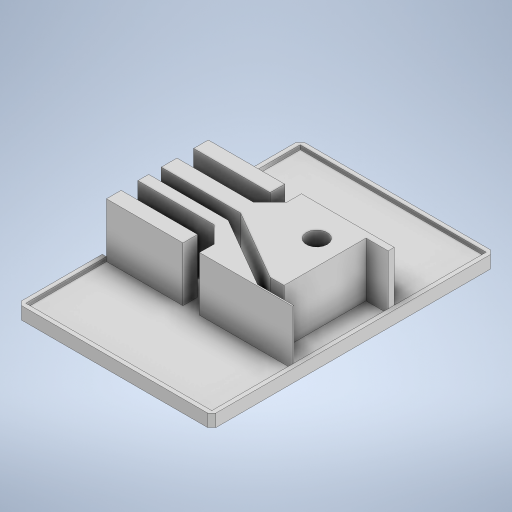
# Autodesk Inventor part: Suporte
Saved by Autodesk Inventor 2024 (Build 280153020, 153B)
## iProperties
Created: 2023-05-31
Part Number: Suporte
Material: Genérico
Document SubType Name: Modeling
Designer: victo
Density: 1 g/cm^3
Appearance: Padrão
Author: victo
Autodesk Inventor part; units mm, degrees
ref_plane "YZ Plane" through (0, 0, 0) normal (1, 0, 0) x (0, 1, 0)
ref_plane "XZ Plane" through (0, 0, 0) normal (0, 1, 0) x (-1, 0, 0)
ref_plane "XY Plane" through (0, 0, 0) normal (0, 0, 1) x (1, 0, 0)
sketch "Esboço1" plane through (0, 0, 0) normal (0, 1, 0) x (-1, 0, 0)
  line L0 (0.0003, 60.0007) -> (0.0003, 29.9998)
  line L1 (0.0003, 29.9998) -> (0.0003, 29.9999)
  line L2 (-0.9997, 29.9999) -> (-0.9997, 60.0007)
  circle A0 centre (11.1, 41.2) radius 2.5
  line L3 (5.3003, 54.8257) -> (5.3003, 35.2257)
  line L4 (5.3003, 35.2257) -> (0.0003, 35.2257)
  line L5 (0.0003, 29.9999) -> (0.0003, 14.4635)
  line L6 (-0.9997, 14.4635) -> (-0.9997, 29.9999)
  line L7 (44.5003, 33.7635) -> (45.5003, 33.7635)
  line L8 (44.5003, 58.1254) -> (45.5003, 58.1254)
  line L9 (26.2003, 33.7635) -> (26.2003, 37.2635)
  line L10 (26.2003, 37.2635) -> (44.5003, 37.2635)
  line L11 (22.2003, 33.7635) -> (0.0003, 33.7635)
  line L12 (22.2003, 33.7635) -> (22.2003, 37.2635)
  line L13 (26.2003, 33.7635) -> (45.0003, 33.7635)
  line L14 (37.268, 41.2635) -> (44.5003, 41.2635)
  line L15 (22.2003, 37.2635) -> (26.2003, 41.2635)
  line L16 (37.268, 41.2635) -> (26.2003, 41.2635)
  line L17 (43.0622, 54.6254) -> (44.5003, 54.6254)
  line L18 (43.0622, 54.6254) -> (26.2003, 54.6254)
  line L19 (26.2003, 54.6254) -> (26.2003, 58.1254)
  line L20 (22.2003, 54.6254) -> (22.2503, 58.1254)
  line L21 (26.2003, 50.6254) -> (22.2003, 54.6254)
  line L22 (26.2003, 50.6254) -> (44.5003, 50.6254)
  line L23 (5.3003, 54.8257) -> (8.6381, 54.8257)
  line L24 (8.6381, 57.8257) -> (0.0003, 57.8257)
  line L25 (44.5003, 45.0257) -> (25.488, 45.0257)
  line L26 (25.488, 48.0257) -> (44.5003, 48.0257)
  line L27 (8.6381, 57.8257) -> (25.488, 48.0257)
  line L28 (8.6381, 54.8257) -> (25.488, 45.0257)
  line L29 (0.0003, 58.1254) -> (22.2503, 58.1254)
  line L30 (26.2003, 58.1254) -> (44.5003, 58.1254)
  line L31 (44.5003, 54.6254) -> (44.5003, 58.1254)
  line L32 (44.5003, 48.0257) -> (44.5003, 50.6254)
  line L33 (44.5003, 33.7635) -> (44.5003, 37.2635)
  line L34 (44.5003, 41.2635) -> (44.5003, 45.0257)
  line L35 (44.5003, 37.2635) -> (44.5003, 41.2635)
  line L36 (44.5003, 45.0257) -> (44.5003, 48.0257)
  line L37 (44.5003, 50.6254) -> (44.5003, 54.6254)
  line L38 (44.5003, 33.968) -> (44.5003, 11.768)
  line L39 (44.5003, 11.768) -> (0.0003, 11.768)
  line L40 (0.0003, 11.768) -> (0.0003, 14.4635)
  line L41 (45.5003, 33.7635) -> (45.5003, 11.768)
  line L42 (44.5003, 58.1254) -> (44.5003, 77.4254)
  line L43 (44.5003, 77.4254) -> (0.0003, 77.4254)
  line L44 (0.0003, 60.0007) -> (0.0003, 77.4254)
  line L45 (45.5003, 58.1254) -> (45.5003, 77.4254)
  line L46 (45.5003, 77.4254) -> (44.5003, 78.4254)
  line L47 (0.0003, 78.4254) -> (-0.9997, 77.4254)
  line L48 (0.0003, 78.4254) -> (44.5003, 78.4254)
  line L49 (-0.9997, 60.0007) -> (-0.9997, 77.4254)
  line L50 (0.0003, 10.768) -> (-0.9997, 11.768)
  line L51 (45.5003, 11.768) -> (44.5003, 10.768)
  line L52 (-0.9997, 11.768) -> (-0.9997, 14.4635)
  line L53 (0.0003, 10.768) -> (44.5003, 10.768)
  point P0 (0, 0)
  dimension "d40" = 1
  dimension "d64" = 5
  dimension "d76" = 19.6
  dimension "d86" = 44.5
  dimension "d90" = 1
  dimension "d91" = 1
  dimension "d94" = 4
  dimension "d102" = 3
  dimension "d103" = 3
  dimension "d116" = 22.2
  dimension "d118" = 19.3
  constraints: 108 end point, 26 perpendicular, 10 point on line, 9 horizontal, 9 vertical, 4 collinear, 2 parallel, 1 centre point, 1 midpoint
  measures "d40" distance of L1.end L2.start
  measures "d64" diameter of A0
  measures "d76" distance of L3.start L3.end
  measures "d86" distance of L29.start L8.start
  measures "d90" distance of L7.start L7.end
  measures "d91" distance of L8.start L8.end
  measures "d94" distance of L9.start L11.start
  measures "d102" distance of L23.end L24.start
  measures "d103" distance of L25.end L26.start
  measures "d116" distance of L38.start L38.end
  measures "d118" distance of L31.end L42.end
extrude "Extrusão27" add sketch "Esboço1" along normal blind 3 contours L0 L5 L40 L39 L38 L7 L41 L51 L53 L50 L52 L6 L2 L49 L47 L48 L46 L45 L8 L42 L43 L44
extrude "Extrusão28" add sketch "Esboço1" along normal blind 2 contours L44 L43 L42 L30 L19 L18 L17 L37 L22 L21 L20 L29 L0 | L24 L27 L26 L36 L25 L28 L23 L3 L4 L0 | L11 L12 L15 L16 L14 L35 L10 L9 L13 L38 L39 L40 L5 L0
extrude "Extrusão29" add sketch "Esboço1" along normal blind 15 contours L29 L20 L21 L22 L32 L26 L27 L24 L0 | L4 L3 L23 L28 L25 L34 L14 L16 L15 L12 L11 L0 | L31 L17 L18 L19 L30 | L33 L13 L9 L10
